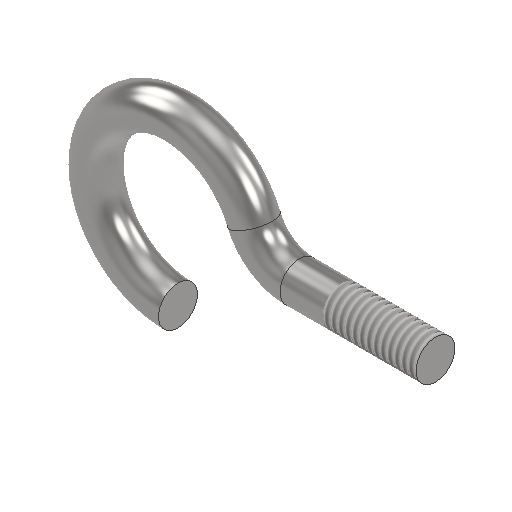
# Autodesk Inventor part: Gancho
Saved by Autodesk Inventor 2026.1 (Build 301233000, 233)
## iProperties
Created: 2025-08-11
Part Number: Gancho
Material: Acero inoxidable
Document SubType Name: Modeling
Designer: gianm
Density: 8 g/cm^3
Appearance: Semipulido
Author: gianm
Autodesk Inventor part; units mm, degrees
ref_plane "YZ Plane" through (0, 0, 0) normal (1, 0, 0) x (0, 1, 0)
ref_plane "XZ Plane" through (0, 0, 0) normal (0, 1, 0) x (-1, 0, 0)
sketch "Boceto1" plane through (0, 0, 0) normal (0, 0, 1) x (1, 0, 0)
  arc A0 (6.0272, 2.4337) -> (0, -6.5) centre (0, 0) ccw
  arc A1 (6.0272, 2.4337) -> (7.7817, 1.25) centre (7.7817, 3.1421) ccw
  line L0 (7.7817, 1.25) -> (16.5, 1.25)
  line L1 (16.5, 1.25) -> (16.5, -1.25) construction
  line L2 (16.5, 0) -> (-6.5, 0) construction
  dimension "d0" = 2.5
  dimension "d9" = 6.5
  dimension "d10" = 23
  constraints: 6 end point, 5 point on circle, 2 centre point, 2 horizontal, 2 tangent, 1 coincident, 1 midpoint, 1 point on line, 1 vertical, 1 vertical alignment
  measures "d0" distance of L0.end L1.end
  measures "d9" radius of A0
  measures "d10" distance of L2.end L2.start
ref_plane "Plano de trabajo1" through (16.5, 1.25, 0) normal (1, 0, 0) x (0, 1, 0)
sketch "Boceto3" plane through (16.5, 1.25, 0) normal (1, 0, 0) x (0, 1, 0)
  circle A0 centre (-1.25, 0) radius 1.25
  point P0 (-1.25, 0)
  constraints: 1 centre point, 1 coincident
sweep "Barrido1" add profiles "Boceto3" path "Boceto1"
thread "Rosca1"
